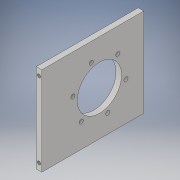
# Autodesk Inventor part: motor mount
Saved by Autodesk Inventor 2019 (Build 230136000, 136)
## iProperties
Created: 2020-09-24
Part Number: motor mount
Material: Generic
Document SubType Name: Modeling
Designer: User
Density: 1 g/cm^3
Appearance: Default
Author: User
Autodesk Inventor part; units mm, degrees
ref_plane "YZ Plane" through (0, 0, 0) normal (1, 0, 0) x (0, 1, 0)
ref_plane "XZ Plane" through (0, 0, 0) normal (0, 1, 0) x (-1, 0, 0)
ref_plane "XY Plane" through (0, 0, 0) normal (0, 0, 1) x (1, 0, 0)
sketch "Sketch1" plane through (0, 0, 0) normal (1, 0, 0) x (0, 1, 0)
  circle A0 centre (0, 0) radius 12.7
  line L0 (25.4, 33.02) -> (-25.4, 33.02)
  line L1 (-25.4, 33.02) -> (-25.4, -25.4)
  line L2 (-25.4, -25.4) -> (25.4, -25.4)
  line L3 (25.4, -25.4) -> (25.4, 33.02)
  dimension "d0" = 25.4
  dimension "d1" = 58.42
  dimension "d4" = 25.4
  dimension "d5" = 25.4
  dimension "d6" = 50.8
  constraints: 8 end point, 2 parallel, 1 centre point, 1 coincident, 1 horizontal, 1 perpendicular
  measures "d0" diameter of A0
  measures "d1" distance of L2.end L0.start
  measures "d4" distance from line of L2 point (0, 0)
  measures "d5" distance from line of point (0, 0) L3
  measures "d6" distance between parallel lines of L3 L1
extrude "Extrusion1" add sketch "Sketch1" along normal blind 3.175
sketch "Sketch2" plane through (0, -25.4, 33.02) normal (0, 0, 1) x (1, 0, 0)
  line L0 (0, 50.8) -> (0, 0) projected
  line L1 (0, 0) -> (3.175, 0) projected
  line L2 (3.175, 50.8) -> (3.175, 0) projected
  line L3 (0, 50.8) -> (3.175, 50.8) projected
  point P0 (0, 25.4)
  point P1 (1.5875, 46.99)
  point P2 (1.5875, 3.81)
  dimension "d9" = 3.175
  dimension "d10" = 1.5875
  dimension "d11" = 1.5875
  dimension "d12" = 3.81
  dimension "d13" = 3.81
  measures "d9" distance of L0.start L2.start
  measures "d10" distance from line of L2 point (1.587, 46.99)
  measures "d11" distance from line of L2 point (1.587, 3.81)
  measures "d12" distance from line of point (1.587, 3.81) L1
  measures "d13" distance from line of L3 point (1.587, 46.99)
hole "Hole1" at (1.5875, 21.59, 33.02) at (1.5875, -21.59, 33.02) direction (0, 0, -1) diameter 1.9304 depth 7.6708 tip angle 118
sketch "Sketch3" plane through (3.175, 0, 0) normal (1, 0, 0) x (0, 0, -1)
  point P0 (0, 0)
  point P1 (10.4798, 11.5154)
  point P2 (-4.7327, 14.8335)
  point P3 (-15.2125, 3.3181)
  point P4 (-10.4798, -11.5154)
  point P5 (4.7327, -14.8335)
  point P6 (15.2125, -3.3181)
  dimension "d21" = 15.5702
  dimension "d24" = 360
  constraints: 7 other
  measures "d21" distance of point (0, 0) point (10.48, 11.515)
hole "Hole2" at (3.175, 11.5154, -10.4798) at (3.175, 14.8335, 4.7327) at (3.175, 3.3181, 15.2125) at (3.175, -11.5154, 10.4798) at (3.175, -14.8335, -4.7327) at (3.175, -3.3181, -15.2125) direction (-1, 0, 0) diameter 2.3368 end through all
equation "\"d10\" = 0.5 * d9"
equation "\"d11\" = d10"
equation "\"d13\" = d12"
body "Solid1"
